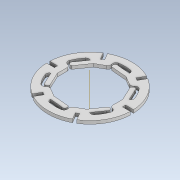
# Autodesk Inventor part: main_ring
Saved by Autodesk Inventor 2020 (Build 240168000, 168)
## iProperties
Created: 2020-09-10
Part Number: main_ring
Material: Generic
Document SubType Name: Modeling
Designer: Admin
Density: 1 g/cm^3
Appearance: Default
Author: Admin
Autodesk Inventor part; units mm, degrees
ref_plane "YZ Plane" through (0, 0, 0) normal (1, 0, 0) x (0, 1, 0)
ref_plane "XZ Plane" through (0, 0, 0) normal (0, 1, 0) x (-1, 0, 0)
ref_plane "XY Plane" through (0, 0, 0) normal (0, 0, 1) x (1, 0, 0)
sketch "Sketch1" plane through (0, 0, 0) normal (0, 1, 0) x (-1, 0, 0)
  circle A0 centre (0, 0) radius 26.5
  circle A1 centre (0, 0) radius 16.5
  dimension "d0" = 53
  dimension "d1" = 33
  constraints: 2 centre point, 2 coincident
  measures "d0" diameter of A0
  measures "d1" diameter of A1
extrude "Extrusion1" add sketch "Sketch1" along normal blind 2
sketch "Sketch2" plane through (0, 2, 0) normal (0, 1, 0) x (1, 0, 0)
  line L0 (-27.5, -1) -> (-21.5, -1)
  line L1 (-21.5, -1) -> (-21.5, 1)
  line L2 (-21.5, 1) -> (-27.5, 1)
  line L3 (-27.5, 1) -> (-27.5, -1)
  circle A0 centre (0, 0) radius 26.5 projected
  point P0 (-26.4811, 1)
  point P1 (-26.4811, -1)
  dimension "d4" = 1
  dimension "d5" = 6
  dimension "d6" = 2
  dimension "d7" = 21.5
  constraints: 8 end point, 2 parallel, 1 horizontal, 1 perpendicular
  measures "d4" distance from line of point (0, 0) L0
  measures "d5" distance of L0.start L0.end
  measures "d6" distance of L2.end L0.start
  measures "d7" distance from line of point (0, 0) L1
extrude "Extrusion2" cut sketch "Sketch2" against normal blind 2 contours A0 L2 L1 L0 picked at (-23.166, -0.1111)
pattern_circular "Circular Pattern1" count 6 over 360 about axis through (0, -10, 0) along (0, 1, 0) of "Extrusion2"
sketch "Sketch3" plane through (0, 2, 0) normal (0, 1, 0) x (1, 0, 0)
  line L0 (-21.5, -5) -> (-17.5, -5)
  line L1 (-17.5, -5) -> (-17.5, 5)
  line L2 (-17.5, 5) -> (-21.5, 5)
  line L3 (-21.5, 1) -> (-21.5, -1) projected
  line L4 (-26.4811, 1) -> (-21.5, 1) projected
  line L5 (-21.5, -1) -> (-26.4811, -1) projected
  arc A0 (-21.5, -5) -> (-19.1164, -11.0369) centre (0, 0) ccw
  arc A1 (-19.1164, 11.0369) -> (-21.5, 5) centre (0, 0) ccw
  line L6 (-19.1164, -11.0369) -> (0, 0)
  line L7 (0, 0) -> (-19.1164, 11.0369)
  line L8 (-37.0736, 0) -> (37.0736, 0) projected
  dimension "d14" = 4
  dimension "d15" = 4
  dimension "d16" = 4
  dimension "d17" = 4
  dimension "d18" = 4
  dimension "d19" = 30
  dimension "d20" = 30
  constraints: 10 end point, 4 point on circle, 2 centre point, 2 coincident, 2 perpendicular, 1 horizontal
  measures "d14" distance between parallel lines of L1 L3
  measures "d15" distance between parallel lines of L4 L2
  measures "d16" distance between parallel lines of L5 L0
  measures "d17" distance of L0.start L0.end
  measures "d18" distance of L1.end L2.end
  measures "d19" angle of L8 L6
  measures "d20" angle of L8 L7
extrude "Extrusion3" cut sketch "Sketch3" against normal blind 2
pattern_circular "Circular Pattern2" count 6 over 360 about axis through (0, -10, 0) along (0, 1, 0) of "Extrusion3"
fillet "Fillet1" radius 2 24 edges at (-17.5, 1, 5) (-17.5, 1, -5) (-21.5, 1, -5) (-21.5, 1, 5) (-4.4199, 1, 17.6554) (-13.0801, 1, -12.6554) (-6.4199, 1, -21.1195) (-4.4199, 1, -17.6554) (13.0801, 1, -12.6554) (4.4199, 1, -17.6554) (17.5, 1, 5) (13.0801, 1, 12.6554) (21.5, 1, -5) (17.5, 1, -5) (4.4199, 1, 17.6554) (6.4199, 1, 21.1195) (15.0801, 1, 16.1195) (21.5, 1, 5) (6.4199, 1, -21.1195) (-15.0801, 1, -16.1195) (-13.0801, 1, 12.6554) (-15.0801, 1, 16.1195) (-6.4199, 1, 21.1195) (15.0801, 1, -16.1195)
sketch "Sketch4" plane through (0, 2, 0) normal (0, 1, 0) x (1, 0, 0)
  arc A0 (-19.1672, -4.9721) -> (-17.5, -3) centre (-19.5, -3) ccw projected
  arc A1 (-16.3706, -12) -> (-13.3706, -12) centre (-14.8706, -12) ccw
  line L0 (-13.3706, -12) -> (-18.5, -1)
  line L1 (-18.5, -1) -> (-21.5, -1)
  line L2 (-21.5, -1) -> (-16.3706, -12)
  line L3 (-21.5, -1) -> (-26.4811, -1) projected
  point P0 (0, 0)
  dimension "d9" = 0
  dimension "d31" = 3
  dimension "d32" = 1.5
  dimension "d33" = 115
  dimension "d34" = 11
  dimension "d35" = 0
  dimension "d36" = 11
  constraints: 6 end point, 2 point on circle, 1 centre point, 1 parallel
  measures "d31" distance of L1.end L0.end
  measures "d32" radius of A1
  measures "d33" angle of L2 L3
  measures "d34" vertical distance of L0.start L0.end
  measures "d35" vertical distance of L1.end L0.end
  measures "d36" distance from line of L3 A1.centre
extrude "Extrusion4" add sketch "Sketch4" against normal blind 2
pattern_circular "Circular Pattern3" count 6 over 360 about axis through (0, -10, 0) along (0, 1, 0) of "Extrusion4"
body "Solid1"
